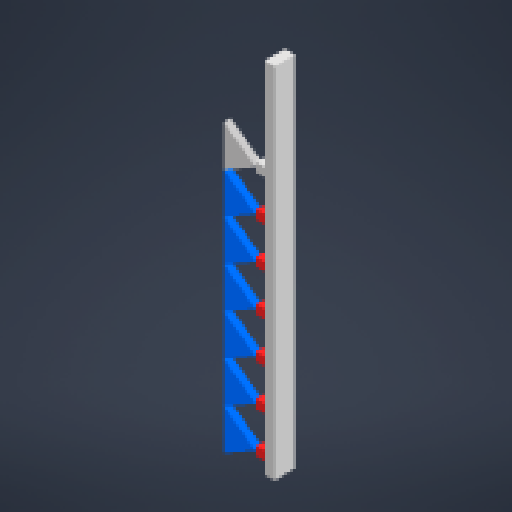
# Autodesk Inventor part: ДМФ 081 труба форсунки v2.0
Saved by Autodesk Inventor 2026.2 (Build 302298010, 298A)
## iProperties
Created: 2024-06-28
Part Number: ДМФ 081 труба форсунки v2.0
Material: Generic
Document SubType Name: Modeling
Designer: admin
Density: 1 g/cm^3
Appearance: Default
Author: admin
Autodesk Inventor part; units mm, degrees
ref_plane "YZ Plane" through (0, 0, 0) normal (1, 0, 0) x (0, 1, 0)
ref_plane "XZ Plane" through (0, 0, 0) normal (0, 1, 0) x (-1, 0, 0)
ref_plane "XY Plane" through (0, 0, 0) normal (0, 0, 1) x (1, 0, 0)
sketch "Sketch2" plane through (0, 0, 0) normal (0, 0, 1) x (1, 0, 0)
  line L0 (-10, 20) -> (10, 20)
  line L1 (10, 20) -> (10, -20)
  line L2 (10, -20) -> (-10, -20)
  line L3 (-10, -20) -> (-10, 20)
  line L4 (-10, 20) -> (10, -20) construction
  line L5 (10, 20) -> (-10, -20) construction
  point P0 (0, 0)
  dimension "d8" = 20
  dimension "d9" = 40
  constraints: 12 end point, 2 midpoint, 2 parallel, 1 horizontal, 1 perpendicular
  measures "d8" distance of L1.end L2.end
  measures "d9" distance of L0.end L1.end
extrude "Extrusion2" add sketch "Sketch2" against normal blind 700
sketch "Sketch3" plane through (0, 0, 0) normal (0, 1, 0) x (-1, 0, 0)
  line L0 (10, 0) -> (-10, 0) construction
  line L1 (10, 0) -> (10, -700) construction
  line L2 (-10, -700) -> (10, -700) construction
  line L3 (-10, 0) -> (-10, -700) construction
  line L4 (10, -680) -> (35, -680)
  line L5 (35, -680) -> (35, -695)
  line L6 (35, -695) -> (10, -695)
  line L7 (10, -695) -> (10, -680)
  line L8 (35, -687.5) -> (99.3571, -687.5)
  line L9 (35, -687.5) -> (99.3571, -646.5)
  line L10 (35, -687.5) -> (99.3571, -728.5)
  line L11 (99.3571, -728.5) -> (99.3571, -646.5)
  point P0 (0, 0)
  dimension "d21" = 25
  dimension "d22" = 15
  dimension "d23" = 5
  dimension "d24" = 65
  dimension "d25" = 82
  dimension "d26" = 64.3571
  dimension "d27" = 109.3571
  constraints: 18 end point, 2 horizontal, 2 midpoint, 2 parallel, 1 perpendicular, 1 point on line, 1 vertical
  measures "d21" distance of L5.end L6.end
  measures "d22" distance between parallel lines of L6 L4
  measures "d23" distance between parallel lines of L2 L6
  measures "d24" angle of L10 L9
  measures "d25" distance of L10.end L9.end
  measures "d26" distance between parallel lines of L5 L11
  measures "d27" distance between parallel lines of L11 L3
extrude "Extrusion3" add sketch "Sketch3" along normal mid plane 14
pattern_linear "Rectangular Pattern1" count 7 spacing 80 along (0, 0, 1) of "Extrusion3"
body "Solid2"
